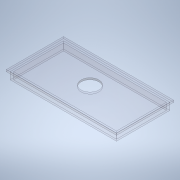
# Autodesk Inventor part: Tapa
Saved by Autodesk Inventor 2021 (Build 250183000, 183)
## iProperties
Created: 2021-06-28
Part Number: Tapa
Material: Plástico PBT
Document SubType Name: Modeling
Designer: artur
Density: 1.31 g/cm^3
Appearance: Transparente - Azul pizarra
Author: artur
Autodesk Inventor part; units mm, degrees
ref_plane "YZ Plane" through (0, 0, 0) normal (1, 0, 0) x (0, 1, 0)
ref_plane "XZ Plane" through (0, 0, 0) normal (0, 1, 0) x (-1, 0, 0)
ref_plane "XY Plane" through (0, 0, 0) normal (0, 0, 1) x (1, 0, 0)
sketch "Boceto1" plane through (0, 0, 0) normal (0, 1, 0) x (-1, 0, 0)
  line L0 (0, 0) -> (312, 0)
  line L1 (312, 0) -> (312, 162)
  line L2 (312, 162) -> (0, 162)
  line L3 (0, 162) -> (0, 0)
  circle A0 centre (156, 81) radius 25
  dimension "d0" = 312
  dimension "d1" = 162
  dimension "d20" = 50
  constraints: 8 end point, 2 parallel, 1 centre point, 1 horizontal, 1 perpendicular
  measures "d0" distance of L1.end L2.end
  measures "d1" distance of L0.end L1.end
  measures "d20" diameter of A0
extrude "Extrusión1" add sketch "Boceto1" along normal blind 5
sketch "Boceto2" plane through (0, 0, 0) normal (0, 1, 0) x (-1, 0, 0)
  line L0 (5.5, 5.5) -> (306.5, 5.5)
  line L1 (306.5, 5.5) -> (306.5, 156.5)
  line L2 (306.5, 156.5) -> (5.5, 156.5)
  line L3 (5.5, 156.5) -> (5.5, 5.5)
  line L4 (0, 0) -> (312, 0) projected
  line L5 (312, 0) -> (312, 162) projected
  line L6 (156, 0) -> (156, 97.9426) construction
  line L7 (306.5, 81) -> (119.0739, 81) construction
  line L8 (0, 162) -> (0, 0) construction
  line L9 (10.5, 151.5) -> (301.5, 151.5)
  line L10 (301.5, 151.5) -> (301.5, 10.5)
  line L11 (301.5, 10.5) -> (10.5, 10.5)
  line L12 (10.5, 10.5) -> (10.5, 151.5)
  dimension "d8" = 301
  dimension "d9" = 151
  dimension "d12" = 5.5
  dimension "d13" = 5.5
  dimension "d14" = 5
  dimension "d15" = 5
  dimension "d16" = 5
  dimension "d17" = 5
  constraints: 20 end point, 4 parallel, 3 horizontal, 2 midpoint, 2 perpendicular, 1 vertical
  measures "d8" distance of L0.start L0.end
  measures "d9" distance of L0.end L1.end
  measures "d12" distance between parallel lines of L8 L3
  measures "d13" distance between parallel lines of L4 L0
  measures "d14" distance between parallel lines of L0 L11
  measures "d15" distance between parallel lines of L2 L9
  measures "d16" distance between parallel lines of L12 L3
  measures "d17" distance between parallel lines of L1 L10
extrude "Extrusión2" add sketch "Boceto2" against normal blind 20
thread "Rosca1" size "M14x2" class "6H" standard "ANSI Metric M Profile" full length
thread "Rosca2" size "M50x4" class "6H" standard "ANSI Metric M Profile" full length
equation "\"d15\" = d14"
equation "\"d16\" = d14"
equation "\"d17\" = d14"
